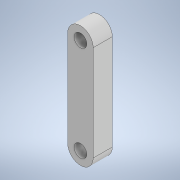
# Autodesk Inventor part: Gripper 5-3
Saved by Autodesk Inventor 2021 (Build 250183000, 183)
## iProperties
Created: 2022-01-08
Part Number: Gripper 5-3
Material: Generic
Document SubType Name: Modeling
Designer: Łukasz
Density: 1 g/cm^3
Appearance: Default
Author: Łukasz
Autodesk Inventor part; units mm, degrees
ref_plane "YZ Plane" through (0, 0, 0) normal (1, 0, 0) x (0, 1, 0)
ref_plane "XZ Plane" through (0, 0, 0) normal (0, 1, 0) x (-1, 0, 0)
ref_plane "XY Plane" through (0, 0, 0) normal (0, 0, 1) x (1, 0, 0)
sketch "Sketch1" plane through (0, 0, 0) normal (0, 0, 1) x (1, 0, 0)
  circle A0 centre (0, 0) radius 2
  arc A1 (-4, 0) -> (4, 0) centre (0, 0) ccw
  circle A2 centre (0, 30) radius 2
  arc A3 (4, 30) -> (-4, 30) centre (0, 30) ccw
  line L0 (-4, 0) -> (-4, 30)
  line L1 (4, 30) -> (4, 0)
  dimension "d0" = 4
  dimension "d1" = 8
  dimension "d2" = 4
  dimension "d3" = 8
  dimension "d6" = 30
  constraints: 4 centre point, 4 end point, 4 point on circle, 3 coincident, 2 tangent
  measures "d0" diameter of A0
  measures "d1" diameter of A1
  measures "d2" diameter of A2
  measures "d3" diameter of A3
  measures "d6" distance of A0.centre A2.centre
extrude "Extrusion1" add sketch "Sketch1" along normal blind 6
body "Solid1"
